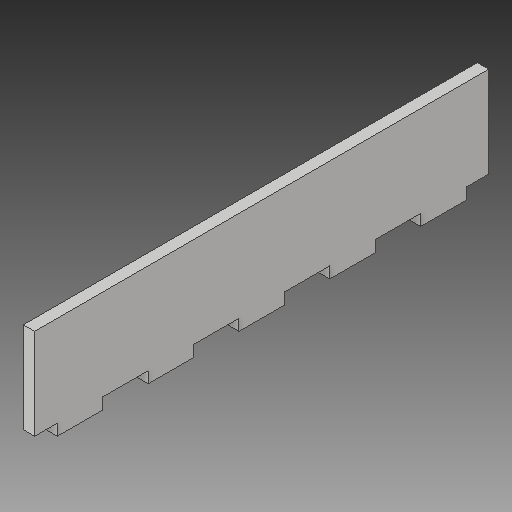
# Autodesk Inventor part: Part5
Saved by Autodesk Inventor 2018 (Build 220112000, 112)
## iProperties
Created: 2018-05-22
Part Number: Part5
Material: Generic
Document SubType Name: Modeling
Designer: Administrator
Density: 1 g/cm^3
Appearance: Default
Mass: 10.882 g
Surface Area: 79.2337 cm^2
Volume: 10.882 cm^3
Author: Administrator
Autodesk Inventor part; units mm, degrees
ref_plane "YZ Plane" through (0, 0, 0) normal (1, 0, 0) x (0, 1, 0)
ref_plane "XZ Plane" through (0, 0, 0) normal (0, 1, 0) x (-1, 0, 0)
ref_plane "XY Plane" through (0, 0, 0) normal (0, 0, 1) x (1, 0, 0)
sketch "Sketch1" plane through (0, 0, 0) normal (1, 0, 0) x (0, 1, 0)
  line L0 (53.664, -52.0596) -> (28.264, -52.0596)
  line L1 (28.264, -52.0596) -> (28.264, -179.0596)
  line L2 (28.264, -179.0596) -> (53.664, -179.0596)
  line L3 (53.664, -179.0596) -> (53.664, -52.0596)
  line L4 (28.264, -58.4096) -> (25.089, -58.4096)
  line L5 (25.089, -58.4096) -> (25.089, -71.1096)
  line L6 (25.089, -71.1096) -> (28.264, -71.1096)
  line L7 (28.264, -71.1096) -> (28.264, -58.4096)
  line L8 (28.264, -83.8096) -> (25.089, -83.8096)
  line L9 (25.089, -83.8096) -> (25.089, -96.5096)
  line L10 (25.089, -96.5096) -> (28.264, -96.5096)
  line L11 (28.264, -96.5096) -> (28.264, -83.8096)
  line L12 (28.264, -109.2096) -> (25.089, -109.2096)
  line L13 (25.089, -109.2096) -> (25.089, -121.9096)
  line L14 (25.089, -121.9096) -> (28.264, -121.9096)
  line L15 (28.264, -121.9096) -> (28.264, -109.2096)
  line L16 (28.264, -134.6096) -> (25.089, -134.6096)
  line L17 (25.089, -134.6096) -> (25.089, -147.3096)
  line L18 (25.089, -147.3096) -> (28.264, -147.3096)
  line L19 (28.264, -147.3096) -> (28.264, -134.6096)
  line L20 (28.264, -160.0096) -> (25.089, -160.0096)
  line L21 (25.089, -160.0096) -> (25.089, -172.7096)
  line L22 (25.089, -172.7096) -> (28.264, -172.7096)
  line L23 (28.264, -172.7096) -> (28.264, -160.0096)
  point P0 (0, 0)
  dimension "d0" = 127
  dimension "d1" = 25.4
  dimension "d2" = 6.35
  dimension "d3" = 3.175
  dimension "d4" = 12.7
  dimension "d5" = 12.7
  dimension "d6" = 12.7
  dimension "d7" = 12.7
  dimension "d8" = 12.7
  dimension "d9" = 12.7
  dimension "d10" = 12.7
  dimension "d11" = 12.7
  dimension "d12" = 12.7
  constraints: 48 end point, 12 parallel, 8 point on line, 6 horizontal, 6 perpendicular
  measures "d0" distance between parallel lines of L2 L0
  measures "d1" distance between parallel lines of L3 L1
  measures "d2" distance between parallel lines of L0 L4
  measures "d3" distance between parallel lines of L1 L5
  measures "d4" distance between parallel lines of L6 L4
  measures "d5" distance between parallel lines of L6 L8
  measures "d6" distance between parallel lines of L10 L8
  measures "d7" distance between parallel lines of L10 L12
  measures "d8" distance between parallel lines of L14 L12
  measures "d9" distance between parallel lines of L16 L14
  measures "d10" distance between parallel lines of L18 L16
  measures "d11" distance between parallel lines of L20 L18
  measures "d12" distance between parallel lines of L22 L20
extrude "Extrusion1" add sketch "Sketch1" along normal blind 3.175
body "Solid1"
